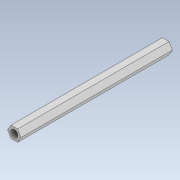
# Autodesk Inventor part: M3-Standoff-51mm
Saved by Autodesk Inventor 2020 (Build 240168000, 168)
## iProperties
Created: 2021-07-13
Part Number: M3-Standoff-51mm
Material: Generic
Document SubType Name: Modeling
Designer: Val
Density: 1 g/cm^3
Appearance: Default
Author: Val
Autodesk Inventor part; units mm, degrees
ref_plane "YZ Plane" through (0, 0, 0) normal (1, 0, 0) x (0, 1, 0)
ref_plane "XZ Plane" through (0, 0, 0) normal (0, 1, 0) x (-1, 0, 0)
ref_plane "XY Plane" through (0, 0, 0) normal (0, 0, 1) x (1, 0, 0)
sketch "Base" plane through (0, 0, 0) normal (0, 0, 1) x (1, 0, 0)
  circle A0 centre (0, 0) radius 1.5 construction
  circle A1 centre (0, 0) radius 2.25 construction
  line L0 (1.125, 1.9486) -> (2.25, 0)
  line L1 (2.25, 0) -> (1.125, -1.9486)
  line L2 (1.125, -1.9486) -> (-1.125, -1.9486)
  line L3 (-1.125, -1.9486) -> (-2.25, 0)
  line L4 (-2.25, 0) -> (-1.125, 1.9486)
  line L5 (-1.125, 1.9486) -> (1.125, 1.9486)
  line L6 (-3.15, 0) -> (3.15, 0) projected
  dimension "d1" = 4.5
  dimension "d0" = 3
  constraints: 12 end point, 3 coincident, 1 centre point, 1 parallel, 16 other
  measures "d0" diameter of A0
extrude "BaseFeature" add sketch "Base" along normal blind 51
sketch "MountHole" plane through (0, 0, 51) normal (0, 0, 1) x (1, 0, 0)
  point P0 (0, 0)
hole "MountHoleFeature" at (0, 0, 51) direction (0, 0, -1) diameter 2.459 end through all thread size "M3x0.5" class "6H" standard "ISO Metric profile"
body "Solid1"
